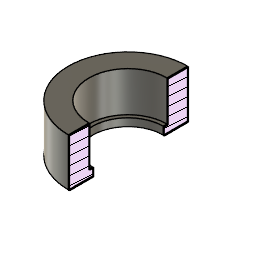
roket mount 1 (Autodesk Fusion 360 design; units mm, degrees)
part number: 2026-05-01-17-17-46-245
Autodesk Fusion 360 part; units mm, degrees
sketch "Sketch1" plane through (0, 0, 0) normal (0, 0, 1) x (1, 0, 0)
  circle A0 centre (0, 0) radius 25
  circle A1 centre (0, 0) radius 14.8
  dimension "d1" = 50
  dimension "d8" = 29.6
  constraint coincident A0.centre A1.centre
  constraint concentric A0 A1
  measures "d1" diameter of A0
  measures "d8" diameter of A1
extrude "Extrude1" add sketch "Sketch1" along normal blind 10 contours A0 | A1
sketch "Sketch2" plane through (0, 0, 10) normal (0, 0, 1) x (-1, 0, 0)
  circle A0 centre (0, 0) radius 25
  circle A1 centre (0, 0) radius 16.375
  dimension "d5" = 32.75
  constraint coincident A0.centre A1.centre
  measures "d5" diameter of A1
extrude "Extrude2" cut sketch "Sketch2" against normal blind 6.75 contours A1
extrude "Extrude3" cut sketch "Sketch1" along normal blind 35 contours A1
extrude "Extrude4" add 1 faces at (21.971, -2.0555, 10) along direction (0, 0, 1) blind 10
